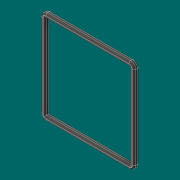
# Autodesk Inventor part: sensorORing
Saved by Autodesk Inventor 2016 (Build 200138000, 138)
## iProperties
Created: 2015-10-19
Part Number: sensorORing
Material: Rubber
Document SubType Name: Modeling
Designer: Sawaiz
Density: 0.93 g/cm^3
Appearance: Rubber - Black
Author: Sawaiz
Autodesk Inventor part; units mm, degrees
ref_plane "YZ Plane" through (0, 0, 0) normal (1, 0, 0) x (0, 1, 0)
ref_plane "XZ Plane" through (0, 0, 0) normal (0, 1, 0) x (-1, 0, 0)
ref_plane "XY Plane" through (0, 0, 0) normal (0, 0, 1) x (1, 0, 0)
sketch "Sketch1" plane through (0, 0, 0) normal (1, 0, 0) x (0, 1, 0)
  line L0 (-26.9875, -26.9875) -> (26.9875, -26.9875)
  line L1 (26.9875, -26.9875) -> (26.9875, 26.9875)
  line L2 (26.9875, 26.9875) -> (-26.9875, 26.9875)
  line L3 (-26.9875, 26.9875) -> (-26.9875, -26.9875)
  line L4 (-26.9875, -26.9875) -> (26.9875, 26.9875) construction
  line L5 (26.9875, -26.9875) -> (-26.9875, 26.9875) construction
  line L6 (-26, -26) -> (26, -26)
  line L7 (26, -26) -> (26, 26)
  line L8 (26, 26) -> (-26, 26)
  line L9 (-26, 26) -> (-26, -26)
  line L10 (-26, -26) -> (26, 26) construction
  line L11 (26, -26) -> (-26, 26) construction
  line L12 (-28.575, -28.575) -> (28.575, -28.575)
  line L13 (28.575, -28.575) -> (28.575, 28.575)
  line L14 (28.575, 28.575) -> (-28.575, 28.575)
  line L15 (-28.575, 28.575) -> (-28.575, -28.575)
  line L16 (-28.575, -28.575) -> (28.575, 28.575) construction
  line L17 (28.575, -28.575) -> (-28.575, 28.575) construction
  point P0 (0, 0)
  dimension "d0" = 53.975
  dimension "d1" = 53.975
  dimension "d2" = 52
  dimension "d3" = 52
  dimension "d4" = 1.5875
  dimension "d5" = 1.5875
  constraints: 36 end point, 6 midpoint, 6 parallel, 3 horizontal, 3 perpendicular
  measures "d0" distance of L2.end L1.end
  measures "d1" distance of L1.end L0.end
  measures "d2" distance of L8.end L7.end
  measures "d3" distance of L7.end L6.end
  measures "d4" distance between parallel lines of L14 L2
  measures "d5" distance between parallel lines of L3 L15
extrude "Extrusion1" add sketch "Sketch1" along normal blind 3.175 contours L3 L2 L1 L0 | L15 L14 L13 L12
fillet "Fillet1" radius 1.0583 16 edges at (3.175, 0, 28.575) (3.175, 0, 26) (0, 0, 28.575) (3.175, 28.575, 0) (3.175, 26, 0) (3.175, -26, 0) (0, -26, 0) (3.175, -28.575, 0) (0, -28.575, 0) (3.175, 0, -26) (0, 0, -26) (3.175, 0, -28.575) (0, 28.575, 0) (0, 0, -28.575) (0, 0, 26) (0, 26, 0)
fillet "Fillet2" radius 3.175 12 edges at (2.865, 28.265, 28.265) (0.31, 28.265, 28.265) (1.5875, 28.575, 28.575) (2.865, 28.265, -28.265) (0.31, 28.265, -28.265) (1.5875, 28.575, -28.575) (1.5875, -28.575, -28.575) (0.31, -28.265, -28.265) (2.865, -28.265, -28.265) (2.865, -28.265, 28.265) (0.31, -28.265, 28.265) (1.5875, -28.575, 28.575)
equation "\"d0\" = sensorHolderSensorWidth"
equation "\"d1\" = sensorHolderSensorHeight"
equation "\"d2\" = detectorWidth"
equation "\"d3\" = detectorHeight"
equation "\"d4\" = 0.5 * oRingWidth"
equation "\"d5\" = 0.5 * oRingWidth"
equation "\"d6\" = sensorHolderORing"
equation "\"d8\" = 0.333333 * oRingWidth"
equation "\"d9\" = oRingWidth"
equation "\"acrylicThickness\" = 6.35"
equation "\"height\" = 101.6"
equation "\"width\" = 101.6"
equation "\"depth\" = 101.6"
equation "\"mirrorAngle\" = 5deg"
equation "\"detectorWidth\" = 52"
equation "\"detectorHeight\" = 52"
equation "\"mirrorThickness\" = 3"
equation "\"fresnelThickness\" = 0.1"
equation "\"focalLength\" = 76.2"
equation "\"ior\" = 1.49"
equation "\"centerThickness\" = 1.524"
equation "\"fresnelAngle\" = 90deg"
equation "\"fresnelEffectiveDiameter\" = 76.2"
equation "\"mirrorSuppourtWidth\" = 38.1"
equation "\"backGrooveBit\" = 4.8006"
equation "\"sensorHolderWidth\" = 88.9"
equation "\"sensorHolderHeight\" = 88.9"
equation "\"sensorHolderSensorHeight\" = 53.975"
equation "\"sensorHolderSensorWidth\" = 53.975"
equation "\"sensorHolderORingGroove\" = 3.175"
equation "\"sensorHolderORing\" = 3.175"
equation "\"sensorHolderFlushORing\" = 3.175"
equation "\"sensorHolderFlushORingID\" = 254"
equation "\"sensorHolderORingID\" = 203.2"
equation "\"oRingWidth\" = 3.175"
equation "\"frontBackORingID\" = 419.1"
equation "\"topBottomHorizontalMirrorGroove\" = 12.7"
equation "\"backMirrorGroove\" = 6.35"
equation "\"mirrorGroove\" = 19.05"
equation "\"mirrorGrooveFillet\" = 6.35"
equation "\"fresnelChamfer\" = 6.35"
equation "\"mirrorGrooveDrill\" = 6.35"
equation "\"mirrorGrooveMill\" = 3.175"
body "Solid1"
